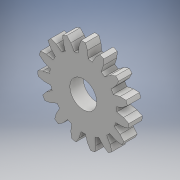
# Autodesk Inventor part: Шестерня
Saved by Autodesk Inventor 2018.1 (Build 221171000, 171)
## iProperties
Part Number: Шестерня
Material: Типовые
Document SubType Name: Modeling
Designer: Пугачева Екатерина
Density: 1 g/cm^3
Appearance: По умолчанию
Author: Пугачева Екатерина
Autodesk Inventor part; units mm, degrees
ref_plane "YZ Plane" through (0, 0, 0) normal (1, 0, 0) x (0, 1, 0)
ref_plane "XZ Plane" through (0, 0, 0) normal (0, 1, 0) x (-1, 0, 0)
ref_plane "XY Plane" through (0, 0, 0) normal (0, 0, 1) x (1, 0, 0)
sketch "Эскиз1" plane through (0, 0, 0) normal (0, 0, 1) x (1, 0, 0)
  line L0 (0, 0) -> (0, 5)
  line L1 (5, 5) -> (17, 5)
  line L2 (17, 5) -> (17, 0)
  line L3 (17, 0) -> (5, 0)
  line L4 (5, 0) -> (5, 5)
  dimension "d0" = 5
  dimension "d1" = 34
  dimension "d2" = 10
  dimension "d3" = 5
  constraints: 10 end point, 2 parallel, 1 horizontal, 1 perpendicular, 1 point on line, 1 vertical
  measures "d0" distance of L0.start L0.end
  measures "d1" diameter of L2 L0
  measures "d2" diameter of L4 L0
  measures "d3" distance of L1.end L2.end
revolve "Вращение1" add sketch "Эскиз1" angle 360 about axis through (0, 0, 0) along (0, 1, 0)
sketch "Эскиз2" plane through (0, 5, 0) normal (0, 1, 0) x (1, 0, 0)
  circle A0 centre (0, 0) radius 12.5 construction
  circle A1 centre (0, 0) radius 15 construction
  circle A2 centre (0, 0) radius 17 projected
  line L0 (-0.785, 12.4753) -> (0.785, 12.4753)
  line L1 (-0.785, 12.4753) -> (-1.57, 14.9176)
  line L2 (0.785, 12.4753) -> (1.57, 14.9176)
  line L3 (-1.57, 14.9176) -> (-2.7475, 16.7765)
  line L4 (1.57, 14.9176) -> (2.7475, 16.7765)
  dimension "d5" = 25
  dimension "d6" = 30
  dimension "d7" = 1.57
  dimension "d8" = 3.14
  dimension "d15" = 5.495
  constraints: 10 end point, 6 point on circle, 2 centre point, 2 coincident, 2 equal length, 1 horizontal
  measures "d5" diameter of A0
  measures "d6" diameter of A1
  measures "d7" distance of L0.start L0.end
  measures "d8" distance of L2.end L1.end
  measures "d15" distance of L4.end L3.end
extrude "Выдавливание1" cut sketch "Эскиз2" against normal up to next contours L4 L2 L0 L1 L3 A2 picked at (-0.2617, 14.1035)
pattern_circular "Круговой массив1" count 15 over 360 about axis through (0, -10, 0) along (0, 1, 0) of "Выдавливание1"
